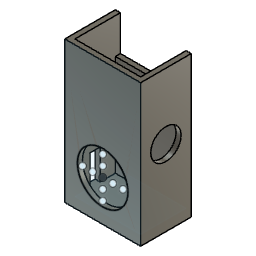
Tree_2piece (Autodesk Fusion 360 design; units mm, degrees)
Autodesk Fusion 360 part; units mm, degrees
note: some values were not read from the file. Set by a fixed rule: which sketch regions a step uses.
sketch "Sketch1" plane through (0, 0, 0) normal (0, 1, 0) x (1, 0, 0) in component "Trunk"
  line L0 (37.5, 70) -> (-37.5, 70)
  line L1 (-37.5, 70) -> (-37.5, -70)
  line L2 (-37.5, -70) -> (37.5, -70)
  line L3 (37.5, -70) -> (37.5, 70)
  line L4 (37.5, 70) -> (-37.5, -70) construction
  line L5 (-37.5, 70) -> (37.5, -70) construction
  line L6 (-37.5, -30) -> (37.5, -30) construction
  dimension "d1" = 75
  dimension "d2" = 140
  dimension "d3" = 100
  constraint horizontal L0
  constraint perpendicular L0 L1
  constraint parallel L0 L2
  constraint parallel L1 L3
  constraint coincident L4 origin
  constraint coincident L5 origin
  constraint coincident L1 L6.start
  constraint perpendicular L1 L6
  constraint coincident L3 L6.end
  measures "d1" distance of L1.end L2.end
  measures "d2" distance of L0.end L1.end
  measures "d3" distance of L0 L6
extrude "Extrude1" add sketch "Sketch1" along normal blind 50 makes body 1 in component "Trunk"
sketch "Sketch2" plane through (0, 50, 0) normal (0, 1, 0) x (-1, 0, 0) in component "Trunk"
  line L0 (-37.5, 70) -> (-37.5, -70)
  line L1 (-37.5, -70) -> (37.5, -70)
  line L2 (37.5, -70) -> (37.5, 70)
  line L3 (37.5, 70) -> (-37.5, 70)
  line L4 (-32.5, -65) -> (32.5, -65)
  line L5 (32.5, -65) -> (32.5, 65)
  line L6 (32.5, 65) -> (-32.5, 65)
  line L7 (-32.5, 65) -> (-32.5, -65)
  line L8 (-32.5, 65) -> (32.5, 65)
  line L9 (32.5, 65) -> (32.5, 70)
  line L10 (32.5, 70) -> (-32.5, 70)
  line L11 (-32.5, 70) -> (-32.5, 65)
  dimension "d6" = -5
  constraint horizontal L8
  constraint vertical L9
  constraint horizontal L10
  constraint vertical L11
  constraint coincident L3 L9.end
extrude "Extrude2" cut sketch "Sketch2" against normal up to surface (45 mm away) contours L3 L6 L8 L9 L10 L11 | L4 L5 L6 L7 L8 bodies 1 in component "Trunk"
sketch "Sketch3" plane through (37.5, 0, 0) normal (1, 0, 0) x (0, 1, 0) in component "Trunk"
  line L0 (0, 70) -> (0, -70)
  line L1 (0, -70) -> (50, -70)
  line L2 (50, -70) -> (50, 70)
  line L3 (50, 70) -> (0, 70)
  circle A0 centre (25, 5) radius 15
  dimension "d9" = 30
  dimension "d10" = 25
  dimension "d11" = 75
  measures "d9" diameter of A0
  measures "d10" distance of L0 A0.centre
  measures "d11" distance of L1 A0.centre
extrude "Extrude3" cut sketch "Sketch3" against normal up to surface (5 mm away) contours A0 bodies 1 in component "Trunk"
sketch "Sketch4" plane through (0, 0, 0) normal (0, 1, 0) x (1, 0, 0) in component "Trunk"
  circle A0 centre (0, 30) radius 25
  line L0 (37.5, 70) -> (-37.5, 70)
  line L1 (-37.5, 70) -> (-37.5, -70)
  dimension "d14" = 50
  dimension "d15" = 40
  dimension "d16" = 37.5
  measures "d14" diameter of A0
  measures "d15" distance of A0.centre L0
  measures "d16" distance of A0.centre L1
extrude "Extrude4" cut sketch "Sketch4" along normal up to surface (5 mm away) bodies 1 in component "Trunk"
sketch "Sketch5" plane through (-37.5, 0, 0) normal (-1, 0, 0) x (0, -1, 0) in component "Trunk"
  line L0 (0, -70) -> (0, 70)
  line L1 (0, 70) -> (-50, 70)
  line L2 (-50, 70) -> (-50, -70)
  line L3 (-50, -70) -> (0, -70)
  line L4 (-20, -65) -> (-30, -65)
  line L5 (-30, -65) -> (-30, -35)
  line L6 (-30, -35) -> (-20, -35)
  line L7 (-20, -35) -> (-20, -65)
  line L8 (-20, -65) -> (-30, -35) construction
  line L9 (-30, -65) -> (-20, -35) construction
  point P0 (-25, -50)
  dimension "d19" = 10
  dimension "d20" = 30
  dimension "d21" = 20
  dimension "d22" = 25
  constraint horizontal L4
  constraint perpendicular L4 L5
  constraint parallel L4 L6
  constraint parallel L5 L7
  constraint coincident L8 P0
  constraint coincident L9 P0
  measures "d19" distance of L5.end L6.end
  measures "d20" distance of L4.end L5.end
  measures "d21" distance of L3 P0
  measures "d22" distance of L2 P0
extrude "Extrude5" cut sketch "Sketch5" against normal up to surface (5 mm away) contours L4 L5 L6 L7 bodies 1 in component "Trunk"
sketch "Sketch7" plane through (9.6288, -5.5064, -65) normal (0, 0, 1) x (-1, 0, 0) in component "Trunk"
  line L0 (42.1288, -10.5064) -> (-22.8712, -10.5064)
  line L1 (-22.8712, -10.5064) -> (-22.8712, -55.5064)
  line L2 (-22.8712, -55.5064) -> (42.1288, -55.5064)
  line L3 (42.1288, -55.5064) -> (42.1288, -35.5064)
  line L4 (42.1288, -35.5064) -> (47.1288, -35.5064)
  line L5 (47.1288, -35.5064) -> (47.1288, -25.5064)
  line L6 (47.1288, -25.5064) -> (42.1288, -25.5064)
  line L7 (42.1288, -25.5064) -> (42.1288, -10.5064)
sketch "Sketch8" plane through (0, 50, 0) normal (0, 1, 0) x (-1, 0, 0) in component "Trunk"
  line L0 (32.5, 70) -> (32.5, -65)
  line L1 (32.5, -65) -> (-32.5, -65)
  line L2 (-32.5, -65) -> (-32.5, 70)
  line L3 (-32.5, 70) -> (-37.5, 70)
  line L4 (-37.5, 70) -> (-37.5, -70)
  line L5 (-37.5, -70) -> (37.5, -70)
  line L6 (37.5, -70) -> (37.5, 70)
  line L7 (37.5, 70) -> (32.5, 70)
  line L8 (-32.5, -65) -> (32.5, -65)
  line L9 (32.5, -65) -> (32.5, 35)
  line L10 (32.5, 35) -> (-32.5, 35)
  line L11 (-32.5, 35) -> (-32.5, -65)
  dimension "d30" = 100
  constraint horizontal L8
  constraint vertical L9
  constraint horizontal L10
  constraint vertical L11
  constraint coincident L1.end L2.start
  measures "d30" distance of L1.end L10.end
extrude "Extrude7" add sketch "Sketch8" against normal blind 5 contours L0 L1 L2 L8 L9 L10 L11 bodies 1 in component "Trunk"
sketch "Sketch9" plane through (0, 50, 0) normal (0, 1, 0) x (-1, 0, 0) in component "Trunk"
  line L0 (32.5, 70) -> (32.5, 35)
  line L1 (32.5, 35) -> (-32.5, 35)
  line L2 (-32.5, 35) -> (-32.5, 70)
  line L3 (-32.5, 70) -> (-37.5, 70)
  line L4 (-37.5, 70) -> (-37.5, -70)
  line L5 (-37.5, -70) -> (37.5, -70)
  line L6 (37.5, -70) -> (37.5, 70)
  line L7 (37.5, 70) -> (32.5, 70)
  circle A0 centre (-27.5, 25) radius 1.5
  circle A1 centre (27.5, 25) radius 1.5
  dimension "d33" = 3
  dimension "d34" = 3
  dimension "d35" = 10
  dimension "d36" = 95
  dimension "d37" = 10
  dimension "d38" = 95
  measures "d33" diameter of A0
  measures "d34" diameter of A1
  measures "d35" distance of L4 A0.centre
  measures "d36" distance of L5 A0.centre
  measures "d37" distance of L6 A1.centre
  measures "d38" distance of L5 A1.centre
extrude "Extrude8" cut sketch "Sketch9" against normal up to surface (5 mm away) contours A0 | A1 bodies 1 in component "Trunk"
sketch "Sketch1 (2)" plane through (0, 0, 0) normal (0, 1, 0) x (1, 0, 0) in component "Leaves"
  line L0 (30, 70) -> (30, -30) construction
  circle A0 centre (-40, -80) radius 50
  line L1 (37.5, 70) -> (-37.5, 70)
  line L2 (0, -1.75) -> (0, -22.5)
  circle A1 centre (40, -80) radius 50
  circle A2 centre (0, -130) radius 50
  dimension "d41" = 100
  dimension "d42" = 100
  dimension "d43" = 150
  dimension "d44" = 40
  dimension "d45" = 100
  dimension "d46" = 100
  dimension "d47" = 150
  dimension "d48" = 40
  dimension "d49" = 200
  constraint vertical L0
  measures "d41" distance of L0.start L0.end
  measures "d42" diameter of A0
  measures "d43" distance of A0.centre L1
  measures "d44" distance of A0.centre L2
  measures "d45" diameter of A1
  measures "d46" diameter of A2
  measures "d47" distance of L1 A1.centre
  measures "d48" distance of L2 A1.centre
  measures "d49" distance of L1 A2.centre
extrude "Extrude1'" add sketch "Sketch1 (2)" along normal blind 60 separate body makes body 2 in component "Leaves"
move_face "OffsetFaces1" offset 10 1 faces at (0, 0, 102.6612) on bodies 2 in component "Leaves"
ref_plane "WorkPlane1" through (0, 0, 10) normal (0, 0, 1) x (1, 0, 0) in component "Leaves"
sketch "Sketch3 (2)" plane through (0, 0, 10) normal (0, 0, 1) x (1, 0, 0) in component "Leaves"
  line L0 (0, 50) -> (40, 50)
  line L1 (40, 50) -> (40, 0)
  line L2 (40, 0) -> (0, 0)
  line L3 (0, 0) -> (0, 50)
  line L4 (0, 50) -> (-40, 50)
  line L5 (-40, 50) -> (-40, 0)
  line L6 (-40, 0) -> (0, 0)
  line L7 (0, 0) -> (0, 50)
  dimension "d54" = 50
  dimension "d55" = 40
  constraint horizontal L0
  constraint vertical L1
  constraint horizontal L2
  constraint vertical L3
  constraint horizontal L4
  constraint vertical L5
  constraint horizontal L6
  constraint vertical L7
  measures "d54" distance of L0.start L2.end
  measures "d55" distance of L0.start L4.end
sketch "Sketch4 (2)" plane through (0, 60, 0) normal (0, 1, 0) x (-1, 0, 0) in component "Leaves"
  arc A0 (0, 50) -> (49.9898, 128.9919) centre (40, 80) ccw
  arc A1 (49.9898, 128.9919) -> (-49.9898, 128.9919) centre (0, 130) ccw
  arc A2 (-49.9898, 128.9919) -> (0, 50) centre (-40, 80) ccw
  arc A3 (45, 35.2786) -> (44.6932, 124.7546) centre (40, 80) ccw
  arc A4 (44.6932, 124.7546) -> (-44.6932, 124.7546) centre (0, 130) ccw
  arc A5 (-44.6932, 124.7546) -> (-45, 35.2786) centre (-40, 80) ccw
  arc A6 (0, 59.3845) -> (44.6932, 124.7546) centre (40, 80) ccw
  arc A7 (44.6932, 124.7546) -> (-44.6932, 124.7546) centre (0, 130) ccw
  arc A8 (-44.6932, 124.7546) -> (0, 59.3845) centre (-40, 80) ccw
  dimension "d59" = -5
  constraint concentric A0 A3
  constraint concentric A1 A4
  constraint concentric A2 A5
extrude "Extrude3'" cut sketch "Sketch4 (2)" against normal up to surface (65 mm away) contours A3 A4 A5 A6 A7 A8 bodies 2 in component "Leaves"
extrude "Extrude2'" cut sketch "Sketch3 (2)" along normal blind 75 bodies 2 in component "Leaves"
sketch "Sketch5 (2)" plane through (0, -5, 0) normal (0, 1, 0) x (-1, 0, 0) in component "Leaves"
  arc A0 (0, 59.3845) -> (44.6932, 124.7546) centre (40, 80) ccw
  arc A1 (44.6932, 124.7546) -> (-44.6932, 124.7546) centre (0, 130) ccw
  arc A2 (-44.6932, 124.7546) -> (0, 59.3845) centre (-40, 80) ccw
  line L0 (47.5, 72.5) -> (-47.5, 72.5)
  line L1 (-47.5, 72.5) -> (-47.5, 77.5)
  line L2 (-47.5, 77.5) -> (47.5, 77.5)
  line L3 (47.5, 77.5) -> (47.5, 72.5)
  line L4 (47.5, 72.5) -> (-47.5, 77.5) construction
  line L5 (-47.5, 72.5) -> (47.5, 77.5) construction
  point P0 (0, 75)
  dimension "d62" = 95
  dimension "d63" = 5
  dimension "d64" = 75
  constraint horizontal L0
  constraint perpendicular L0 L1
  constraint parallel L0 L2
  constraint parallel L1 L3
  constraint coincident L4 P0
  constraint coincident L5 P0
  constraint vertical origin P0
  measures "d62" distance of L1.end L2.end
  measures "d63" distance of L0.end L1.end
  measures "d64" distance of origin P0
extrude "Extrude4'" add sketch "Sketch5 (2)" along normal blind 65 contours L0 L1 L2 L3 bodies 2 in component "Leaves"
sketch "Sketch7 (2)" plane through (0, 0, 72.5) normal (0, 0, -1) x (1, 0, 0) in component "Leaves"
  line L0 (47.5, 5) -> (-47.5, 5)
  line L1 (-47.5, 5) -> (-47.5, -60)
  line L2 (-47.5, -60) -> (47.5, -60)
  line L3 (47.5, -60) -> (47.5, 5)
  line L4 (-47.5, 5) -> (-40, 5)
  line L5 (-40, 5) -> (-40, -60)
  line L6 (-40, -60) -> (-47.5, -60)
  line L7 (-47.5, -60) -> (-47.5, 5)
  line L8 (47.5, -60) -> (40, -60)
  line L9 (40, -60) -> (40, 5)
  line L10 (40, 5) -> (47.5, 5)
  line L11 (47.5, 5) -> (47.5, -60)
  dimension "d76" = 7.5
  dimension "d77" = 7.5
  constraint horizontal L4
  constraint vertical L5
  constraint horizontal L6
  constraint vertical L7
  constraint coincident L2 L5.end
  constraint coincident L0.end L1.start
  constraint horizontal L8
  constraint vertical L9
  constraint horizontal L10
  constraint vertical L11
  constraint coincident L2.end L3.start
  measures "d76" distance of L0.end L4.end
  measures "d77" distance of L2.end L8.end
extrude "Extrude6" add sketch "Sketch7 (2)" along normal blind 40 contours L0 L2 L3 L8 L9 L10 L11 | L0 L1 L2 L4 L5 L6 L7 bodies 2 in component "Leaves"
sketch "Sketch10" plane through (0, -10, 0) normal (0, -1, 0) x (1, 0, 0) in component "Leaves"
  arc A0 (49.9898, 128.9919) -> (-49.9898, 128.9919) centre (0, 130) ccw
  arc A1 (-49.9898, 128.9919) -> (0, 50) centre (-40, 80) ccw
  arc A2 (0, 50) -> (49.9898, 128.9919) centre (40, 80) ccw
  line L0 (35.5, 91) -> (-35.5, 91)
  line L1 (-35.5, 91) -> (-35.5, 114)
  line L2 (-35.5, 114) -> (35.5, 114)
  line L3 (35.5, 114) -> (35.5, 91)
  line L4 (35.5, 91) -> (-35.5, 114) construction
  line L5 (-35.5, 91) -> (35.5, 114) construction
  line L6 (47.5, 77.5) -> (-47.5, 77.5)
  point P0 (0, 102.5)
  dimension "d89" = 71
  dimension "d90" = 23
  dimension "d91" = 25
  constraint horizontal L0
  constraint perpendicular L0 L1
  constraint parallel L0 L2
  constraint parallel L1 L3
  constraint coincident L4 P0
  constraint coincident L5 P0
  measures "d89" distance of L1.end L2.end
  measures "d90" distance of L0.end L1.end
  measures "d91" distance of P0 L6
extrude "Extrude9" cut sketch "Sketch10" against normal up to surface (5 mm away) contours L0 L1 L2 L3 bodies 2 in component "Leaves"
sketch "Sketch11" plane through (-0.8027, -10, 3.4654) normal (0, -1, 0) x (1, 0, 0) in component "Leaves"
  line L0 (36.3027, 110.5346) -> (36.3027, 87.5346)
  line L1 (36.3027, 87.5346) -> (-34.6973, 87.5346)
  line L2 (-34.6973, 87.5346) -> (-34.6973, 110.5346)
  line L3 (-34.6973, 110.5346) -> (36.3027, 110.5346)
  arc A0 (50.7925, 125.5264) -> (-49.1872, 125.5264) centre (0.8027, 126.5346) ccw
  arc A1 (-49.1872, 125.5264) -> (0.8027, 46.5346) centre (-39.1973, 76.5346) ccw
  arc A2 (0.8027, 46.5346) -> (50.7925, 125.5264) centre (40.8027, 76.5346) ccw
  circle A3 centre (-63.6973, 70) radius 6.5
  line L4 (71.8027, 60) -> (58.8027, 60)
  line L5 (58.8027, 60) -> (58.8027, 80)
  line L6 (58.8027, 80) -> (71.8027, 80)
  line L7 (71.8027, 80) -> (71.8027, 60)
  line L8 (71.8027, 60) -> (58.8027, 80) construction
  line L9 (58.8027, 60) -> (71.8027, 80) construction
  point P0 (65.3027, 70)
  dimension "d94" = 13
  dimension "d95" = 13
  dimension "d96" = 20
  dimension "d97" = 29
  dimension "d98" = 29
  constraint horizontal L4
  constraint perpendicular L4 L5
  constraint parallel L4 L6
  constraint parallel L5 L7
  constraint coincident L8 P0
  constraint coincident L9 P0
  measures "d94" diameter of A3
  measures "d95" distance of L5.end L6.end
  measures "d96" distance of L4.end L5.end
  measures "d97" distance of L2 A3.centre
  measures "d98" distance of L0 P0
extrude "Extrude10" cut sketch "Sketch11" against normal up to surface (5 mm away) contours A3 | L4 L5 L6 L7 bodies 2 in component "Leaves"
sketch "Sketch12" plane through (0, -5, 0) normal (0, 1, 0) x (-1, 0, 0) in component "Leaves"
  circle A0 centre (64.5, 73.4654) radius 6.5
  line L0 (-71, 63.4654) -> (-71, 83.4654)
  line L1 (-71, 83.4654) -> (-58, 83.4654)
  line L2 (-58, 83.4654) -> (-58, 63.4654)
  line L3 (-58, 63.4654) -> (-71, 63.4654)
  line L4 (-35.5, 91) -> (-35.5, 114)
  line L5 (-35.5, 114) -> (35.5, 114)
  line L6 (35.5, 114) -> (35.5, 91)
  line L7 (35.5, 91) -> (-35.5, 91)
  line L8 (-47.5, 35.6294) -> (-47.5, 77.5)
  line L9 (-47.5, 77.5) -> (47.5, 77.5)
  line L10 (47.5, 77.5) -> (47.5, 35.6294)
  arc A1 (47.5, 35.6294) -> (44.6932, 124.7546) centre (40, 80) ccw
  arc A2 (44.6932, 124.7546) -> (-44.6932, 124.7546) centre (0, 130) ccw
  arc A3 (-44.6932, 124.7546) -> (-47.5, 35.6294) centre (-40, 80) ccw
  circle A4 centre (-36.5, 117) radius 2
  circle A5 centre (-36.5, 88) radius 2
  circle A6 centre (36.5, 117) radius 2
  circle A7 centre (36.5, 88) radius 2
  dimension "d144" = 4
  dimension "d145" = 4
  dimension "d146" = 4
  dimension "d147" = 3
  dimension "d148" = 1
  dimension "d149" = 1
  dimension "d150" = 3
  dimension "d151" = 3
  dimension "d152" = 1
  dimension "d153" = 4
  dimension "d154" = 1
  dimension "d155" = 3
  measures "d144" diameter of A4
  measures "d145" diameter of A5
  measures "d146" diameter of A6
  measures "d147" distance of L5 A4.centre
  measures "d148" distance of L4 A4.centre
  measures "d149" distance of L4 A5.centre
  measures "d150" distance of L7 A5.centre
  measures "d151" distance of L5 A6.centre
  measures "d152" distance of L6 A6.centre
  measures "d153" diameter of A7
  measures "d154" distance of L6 A7.centre
  measures "d155" distance of L7 A7.centre
extrude "Extrude11" add sketch "Sketch12" along normal blind 2 contours A4 | A5 | A6 | A7 bodies 2 in component "Leaves"
ref_plane "WorkPlane2" through (0, 25, -65) normal (0, 0, -1) x (-1, 0, 0) in component "ShovelHole"
sketch "Sketch2 (2)" plane through (0, 25, -65) normal (0, 0, -1) x (1, 0, 0) in component "ShovelHole"
  line L0 (32.5, 20) -> (-32.5, 20)
  line L1 (-32.5, 20) -> (-32.5, -20)
  line L2 (-32.5, -20) -> (32.5, -20)
  line L3 (32.5, -20) -> (32.5, 20)
  line L4 (32.5, 20) -> (-32.5, -20) construction
  line L5 (-32.5, 20) -> (32.5, -20) construction
  dimension "d123" = 65
  dimension "d124" = 40
  constraint horizontal L0
  constraint perpendicular L0 L1
  constraint parallel L0 L2
  constraint parallel L1 L3
  constraint coincident L4 origin
  constraint coincident L5 origin
  measures "d123" distance of L1.end L2.end
  measures "d124" distance of L0.end L1.end
extrude "Extrude1''" add sketch "Sketch2 (2)" against normal blind 20 separate body makes body 3 in component "ShovelHole"
sketch "Sketch3 (3)" plane through (-32.5, 0, 0) normal (-1, 0, 0) x (0, -1, 0) in component "ShovelHole"
  line L0 (-45, -65) -> (-5, -65)
  line L1 (-5, -65) -> (-5, -45)
  line L2 (-5, -45) -> (-45, -45)
  line L3 (-45, -45) -> (-45, -65)
  line L4 (-43, -63) -> (-7, -63)
  line L5 (-7, -63) -> (-7, -47)
  line L6 (-7, -47) -> (-43, -47)
  line L7 (-43, -47) -> (-43, -63)
  dimension "d127" = -2
extrude "Extrude2''" cut sketch "Sketch3 (3)" against normal up to surface (65 mm away) contours L4 L5 L6 L7 bodies 3 in component "ShovelHole"
sketch "Sketch4 (3)" plane through (0, 0, -45) normal (0, 0, 1) x (-1, 0, 0) in component "ShovelHole"
  line L0 (-32.5, -5) -> (-32.5, -45)
  line L1 (-32.5, -45) -> (32.5, -45)
  line L2 (32.5, -45) -> (32.5, -5)
  line L3 (32.5, -5) -> (-32.5, -5)
  line L4 (0, -30) -> (32.5, -30) construction
  line L5 (32.5, -30) -> (27.5, -30)
  line L6 (27.5, -30) -> (27.5, -20)
  line L7 (27.5, -20) -> (32.5, -20)
  line L8 (32.5, -20) -> (32.5, -30)
  dimension "d135" = 5
  constraint coincident L2 L4.end
  constraint perpendicular L2 L4
  constraint horizontal L5
  constraint vertical L6
  constraint horizontal L7
  constraint vertical L8
  measures "d135" distance of L4.end L5.end
extrude "Extrude3''" cut sketch "Sketch4 (3)" against normal up to surface (2 mm away) contours L2 L5 L6 L7 L8 bodies 3 in component "ShovelHole"
sketch "Sketch5 (3)" plane through (0, 7, 0) normal (0, 1, 0) x (-1, 0, 0) in component "ShovelHole"
  line L0 (-32.5, -47) -> (-32.5, -63)
  line L1 (-32.5, -63) -> (32.5, -63)
  line L2 (32.5, -63) -> (32.5, -47)
  line L3 (32.5, -47) -> (-32.5, -47)
  circle A0 centre (25, -55) radius 2
  dimension "d132" = 4
  dimension "d136" = 8
  dimension "d137" = 7.5
  measures "d132" diameter of A0
  measures "d136" distance of L3 A0.centre
  measures "d137" distance of L2 A0.centre
extrude "Extrude4''" add sketch "Sketch5 (3)" along normal blind 18 contours A0 bodies 3 in component "ShovelHole"
sketch "Sketch1 (3)" plane through (0, 0, -45) normal (0, 0, 1) x (-1, 0, 0)
  line L0 (32.5, -30) -> (27.5, -30)
  line L1 (27.5, -30) -> (27.5, -20)
  line L2 (27.5, -20) -> (32.5, -20)
  line L3 (32.5, -20) -> (32.5, -5)
  line L4 (32.5, -5) -> (-32.5, -5)
  line L5 (-32.5, -5) -> (-32.5, -45)
  line L6 (-32.5, -45) -> (32.5, -45)
  line L7 (32.5, -45) -> (32.5, -30)
  line L8 (-17.5, -16.5) -> (17.5, -16.5)
  line L9 (17.5, -16.5) -> (17.5, -31.5)
  line L10 (17.5, -31.5) -> (-17.5, -31.5)
  line L11 (-17.5, -31.5) -> (-17.5, -16.5)
  line L12 (-17.5, -16.5) -> (17.5, -31.5) construction
  line L13 (17.5, -16.5) -> (-17.5, -31.5) construction
  point P0 (0, -24)
  dimension "d184" = 35
  dimension "d185" = 15
  constraint horizontal L8
  constraint perpendicular L8 L9
  constraint parallel L8 L10
  constraint parallel L9 L11
  constraint coincident L12 P0
  constraint coincident L13 P0
  measures "d184" distance of L9.end L10.end
  measures "d185" distance of L8.end L9.end
extrude "Extrude6'" cut sketch "Sketch1 (3)" against normal up to surface (2 mm away) contours L8 L9 L10 L11 bodies 3 in component "ShovelHole"
sketch "Sketch13" plane through (0, 0, 77.5) normal (0, 0, 1) x (-1, 0, 0) in component "Leaves"
  line L0 (47.5, 5) -> (-47.5, 5)
  line L1 (-47.5, 5) -> (-47.5, -60)
  line L2 (-47.5, -60) -> (47.5, -60)
  line L3 (47.5, -60) -> (47.5, 5)
  circle A0 centre (0, -25) radius 20
  dimension "d156" = 40
  dimension "d157" = 35
  measures "d156" diameter of A0
  measures "d157" distance of L2 A0.centre
extrude "Extrude12" cut sketch "Sketch13" against normal up to surface (5 mm away) contours A0 bodies 2 in component "Leaves"
sketch "Sketch14" plane through (0, 0, 72.5) normal (0, 0, -1) x (1, 0, 0) in component "Leaves"
  circle A0 centre (0, -25) radius 20
  line L0 (40, -60) -> (40, 5)
  line L1 (40, 5) -> (-40, 5)
  line L2 (-40, 5) -> (-40, -60)
  line L3 (-40, -60) -> (40, -60)
  line L4 (-40, -60) -> (40, -60)
  line L5 (40, -60) -> (40, -50)
  line L6 (40, -50) -> (-40, -50)
  line L7 (-40, -50) -> (-40, -60)
  dimension "d160" = 80
  dimension "d161" = 10
  constraint horizontal L4
  constraint vertical L5
  constraint horizontal L6
  constraint vertical L7
  constraint coincident L2.end L3.start
  measures "d160" distance of L2.end L0.start
  measures "d161" distance of L2.end L6.end
extrude "Extrude13" add sketch "Sketch14" along normal blind 60 contours L0 L2 L3 L4 L5 L6 L7 bodies 2 in component "Leaves"
sketch "Sketch15" plane through (0, 50, 0) normal (0, -1, 0) x (1, 0, 0) in component "Leaves"
  line L0 (-40, 72.5) -> (-40, 30)
  line L1 (-40, 30) -> (-40, 12.5)
  line L2 (-40, 12.5) -> (40, 12.5)
  line L3 (40, 12.5) -> (40, 30)
  line L4 (40, 30) -> (40, 72.5)
  line L5 (40, 72.5) -> (-40, 72.5)
  circle A0 centre (-27.5, 25) radius 1.5
  line L6 (-32.5, -65) -> (-32.5, 70)
  line L7 (0, 1.75) -> (0, 22.5)
  circle A1 centre (27.5, 25) radius 1.5
  dimension "d164" = 3
  dimension "d165" = 5
  dimension "d166" = 12.5
  constraint symmetric A0 L7 A1
  measures "d164" diameter of A0
  measures "d165" distance of A0.centre L6
  measures "d166" distance of L2 A0.centre
extrude "Extrude14" cut sketch "Sketch15" against normal up to surface (10 mm away) contours A0 | A1 bodies 2 in component "Leaves"
sketch "Sketch16" plane through (0, 60, 0) normal (0, 1, 0) x (-1, 0, 0) in component "Leaves"
  circle A0 centre (27.5, 25) radius 1.5
  circle A1 centre (-27.5, 25) radius 1.5
  line L0 (-40, 30) -> (-40, 12.5)
  line L1 (-40, 12.5) -> (40, 12.5)
  line L2 (40, 12.5) -> (40, 30)
  arc A2 (40, 30) -> (49.9898, 128.9919) centre (40, 80) ccw
  arc A3 (49.9898, 128.9919) -> (-49.9898, 128.9919) centre (0, 130) ccw
  arc A4 (-49.9898, 128.9919) -> (-40, 30) centre (-40, 80) ccw
  line L3 (-47.5, 77.5) -> (-47.5, 35.6294)
  arc A5 (-44.6932, 124.7546) -> (-47.5, 35.6294) centre (-40, 80) ccw
  arc A6 (44.6932, 124.7546) -> (-44.6932, 124.7546) centre (0, 130) ccw
  arc A7 (47.5, 35.6294) -> (44.6932, 124.7546) centre (40, 80) ccw
  line L4 (47.5, 35.6294) -> (47.5, 77.5)
  line L5 (47.5, 77.5) -> (-47.5, 77.5)
  circle A8 centre (-84.9777, 79.9594) radius 3.5
  circle A9 centre (-84.9777, 79.9594) radius 1.5
  circle A10 centre (0, 175) radius 3.5
  circle A11 centre (0, 175) radius 1.5
  dimension "d169" = 7
  dimension "d170" = -2
  dimension "d171" = 7
  dimension "d172" = -2
  constraint midpoint A6 A10.centre
  measures "d169" diameter of A8
  measures "d171" diameter of A10
extrude "Extrude15" add sketch "Sketch16" against normal blind 10 contours A5 A8 A9 | A5 A9 | A6 A10 A11 | A6 A11 picked at (-84.2514, 82.186) picked at (-84.4907, 79.9594) picked at (-2.2066, 174.2251) picked at (-0.037, 174.4995) bodies 2 in component "Leaves"
mirror "Mirror1" about plane through (0, 0, 0) normal (1, 0, 0) of "Extrude15" in component "Leaves"
sketch "Sketch17" plane through (0, 60, 0) normal (0, 1, 0) x (-1, 0, 0) in component "Leaves"
  arc A0 (44.6932, 124.7546) -> (3.4974, 174.8639) centre (0, 130) ccw
  arc A1 (84.867, 83.4576) -> (44.6932, 124.7546) centre (40, 80) ccw
  arc A2 (84.867, 83.4576) -> (84.8606, 76.4613) centre (84.9777, 79.9594) ccw
  arc A3 (47.5, 35.6294) -> (84.8606, 76.4613) centre (40, 80) ccw
  line L0 (47.5, 35.6294) -> (47.5, 77.5)
  line L1 (47.5, 77.5) -> (-47.5, 77.5)
  line L2 (-47.5, 77.5) -> (-47.5, 35.6294)
  arc A4 (-84.8606, 76.4613) -> (-47.5, 35.6294) centre (-40, 80) ccw
  arc A5 (-84.8606, 76.4613) -> (-84.867, 83.4576) centre (-84.9777, 79.9594) ccw
  arc A6 (-44.6932, 124.7546) -> (-84.867, 83.4576) centre (-40, 80) ccw
  arc A7 (-3.4974, 174.8639) -> (-44.6932, 124.7546) centre (0, 130) ccw
  arc A8 (-3.4974, 174.8639) -> (3.4974, 174.8639) centre (0, 175) ccw
  circle A9 centre (27.5, 25) radius 1.5
  circle A10 centre (-27.5, 25) radius 1.5
  line L3 (-40, 30) -> (-40, 12.5)
  line L4 (-40, 12.5) -> (40, 12.5)
  line L5 (40, 12.5) -> (40, 30)
  arc A11 (40, 30) -> (49.9898, 128.9919) centre (40, 80) ccw
  arc A12 (49.9898, 128.9919) -> (-49.9898, 128.9919) centre (0, 130) ccw
  arc A13 (-49.9898, 128.9919) -> (-40, 30) centre (-40, 80) ccw
  circle A14 centre (-84.9777, 79.9594) radius 1
  circle A15 centre (0, 175) radius 1
  circle A16 centre (84.9777, 79.9594) radius 1
  dimension "d177" = 2
  dimension "d178" = 2
  dimension "d179" = 2
  constraint concentric A5 A14
  constraint concentric A8 A15
  constraint concentric A2 A16
  measures "d177" diameter of A14
  measures "d178" diameter of A15
  measures "d179" diameter of A16
extrude "Extrude16" cut sketch "Sketch17" against normal blind 5 contours A14 | A15 | A16 bodies 2 in component "Leaves"
sketch "Sketch1 (4)" plane through (0, 60, 0) normal (0, 1, 0) x (-1, 0, 0) in component "Lid"
  circle A0 centre (84.9777, 79.9594) radius 1
  circle A1 centre (0, 175) radius 1
  circle A2 centre (-84.9777, 79.9594) radius 1
  arc A3 (44.6932, 124.7546) -> (3.4974, 174.8639) centre (0, 130) ccw
  arc A4 (84.867, 83.4576) -> (44.6932, 124.7546) centre (40, 80) ccw
  arc A5 (84.867, 83.4576) -> (84.8606, 76.4613) centre (84.9777, 79.9594) ccw
  arc A6 (47.5, 35.6294) -> (84.8606, 76.4613) centre (40, 80) ccw
  line L0 (47.5, 35.6294) -> (47.5, 77.5)
  line L1 (47.5, 77.5) -> (-47.5, 77.5)
  line L2 (-47.5, 77.5) -> (-47.5, 35.6294)
  arc A7 (-84.8606, 76.4613) -> (-47.5, 35.6294) centre (-40, 80) ccw
  arc A8 (-84.8606, 76.4613) -> (-84.867, 83.4576) centre (-84.9777, 79.9594) ccw
  arc A9 (-44.6932, 124.7546) -> (-84.867, 83.4576) centre (-40, 80) ccw
  arc A10 (-3.4974, 174.8639) -> (-44.6932, 124.7546) centre (0, 130) ccw
  arc A11 (-3.4974, 174.8639) -> (3.4974, 174.8639) centre (0, 175) ccw
  circle A12 centre (27.5, 25) radius 1.5
  circle A13 centre (-27.5, 25) radius 1.5
  line L3 (-40, 30) -> (-40, 12.5)
  line L4 (-40, 12.5) -> (40, 12.5)
  line L5 (40, 12.5) -> (40, 30)
  arc A14 (40, 30) -> (49.9898, 128.9919) centre (40, 80) ccw
  arc A15 (49.9898, 128.9919) -> (-49.9898, 128.9919) centre (0, 130) ccw
  arc A16 (-49.9898, 128.9919) -> (-40, 30) centre (-40, 80) ccw
  circle A17 centre (0, 130) radius 50
  circle A18 centre (-40, 80) radius 50
  circle A19 centre (40, 80) radius 50
  circle A20 centre (-44, 74) radius 1
  line L6 (0, 20) -> (0, 2.5)
  circle A21 centre (-87.6, 80) radius 1
  circle A22 centre (0, 177.5) radius 1
  circle A23 centre (87.5, 80) radius 1
  circle A24 centre (44, 74) radius 1
  dimension "d188" = 100
  dimension "d189" = 100
  dimension "d190" = 100
  dimension "d191" = 2
  dimension "d192" = 2
  dimension "d193" = 2
  dimension "d194" = 2
  dimension "d195" = 2
  constraint concentric A3 A17
  constraint concentric A7 A18
  constraint concentric A4 A19
  measures "d188" diameter of A17
  measures "d189" diameter of A18
  measures "d190" diameter of A19
  measures "d191" diameter of A20
  measures "d192" diameter of A21
  measures "d193" diameter of A22
  measures "d194" diameter of A23
  measures "d195" diameter of A24
extrude "Extrude1'''" add sketch "Sketch1 (4)" along normal blind 5 separate body contours A0 | A1 | A2 | A3 A4 A17 A18 A19 | A3 A4 A17 A19 | A3 A10 A11 A18 A19 | A3 A10 A11 A15 A17 A18 A19 | A4 A5 A6 L0 L1 A14 A17 A18 A19 | A4 A5 A6 L0 L1 A17 A18 | A9 A10 A17 A18 A19 | A17 A18 A19 | L1 A17 A18 A19 | A9 A10 A17 A18 | L1 L2 A7 A8 A9 A17 A19 | L1 L2 A7 A8 A9 A16 A17 A18 A19 | L1 A18 A19 makes body 4 in component "Lid"
sketch "Sketch1 (5)" plane through (0, 0, 0) normal (0, -1, 0) x (1, 0, 0) in component "SpeakerMesh"
  circle A0 centre (0, -30) radius 25
  line L0 (37.5, -70) -> (37.5, 70)
  line L1 (37.5, 70) -> (-37.5, 70)
  line L2 (-37.5, 70) -> (-37.5, -70)
  line L3 (-37.5, -70) -> (37.5, -70)
  circle A1 centre (0, -30) radius 25
  circle A2 centre (0, -30) radius 1.25
  circle A3 centre (0, -20) radius 1.25
  circle A4 centre (0, -10) radius 1.25
  circle A5 centre (0, -40) radius 1.25
  circle A6 centre (0, -50) radius 1.25
  circle A7 centre (10, -30) radius 1.25
  circle A8 centre (20, -30) radius 1.25
  circle A9 centre (-10, -30) radius 1.25
  circle A10 centre (-20, -30) radius 1.25
  dimension "d198" = 50
  dimension "d199" = 2.5
  dimension "d200" = 2.5
  dimension "d201" = 2.5
  dimension "d202" = 2.5
  dimension "d203" = 2.5
  dimension "d204" = 2.5
  dimension "d205" = 2.5
  dimension "d206" = 2.5
  dimension "d207" = 2.5
  constraint concentric A0 A1
  measures "d198" diameter of A1
  measures "d199" diameter of A2
  measures "d200" diameter of A3
  measures "d201" diameter of A4
  measures "d202" diameter of A5
  measures "d203" diameter of A6
  measures "d204" diameter of A7
  measures "d205" diameter of A8
  measures "d206" diameter of A9
  measures "d207" diameter of A10
component "Leaves" placed x (1, 0, 0) y (0, 1, 0) z (0, 0, 1) at (0, 0, 0)
component "Trunk" placed x (1, 0, 0) y (0, 1, 0) z (0, 0, 1) at (0, 0, 0)
component "ShovelHole" placed x (1, 0, 0) y (0, 1, 0) z (0, 0, 1) at (0, 0, 0)
component "Lid" placed x (1, 0, 0) y (0, 1, 0) z (0, 0, 1) at (0, 0, 0)
component "SpeakerMesh" placed x (1, 0, 0) y (0, 1, 0) z (0, 0, 1) at (0, 0, 0)
